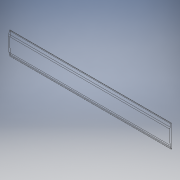
# Autodesk Inventor part: element_1
Saved by Autodesk Inventor 2018.1 (Build 221171000, 171)
## iProperties
Created: 2017-10-22
Part Number: element_1
Material: CFRP
Document SubType Name: Modeling
Designer: ku_sk
Density: 1.43 g/cm^3
Appearance: カーボンファイバー
Mass: 1502.98 g
Surface Area: 2648.54 cm^2
Volume: 1051.04 cm^3
Author: ku_sk
Autodesk Inventor part; units mm, degrees
ref_plane "YZ Plane" through (0, 0, 0) normal (1, 0, 0) x (0, 1, 0)
ref_plane "XZ Plane" through (0, 0, 0) normal (0, 1, 0) x (-1, 0, 0)
ref_plane "XY Plane" through (0, 0, 0) normal (0, 0, 1) x (1, 0, 0)
sketch "スケッチ1" plane through (0, 0, 0) normal (1, 0, 0) x (0, 1, 0)
  line L0 (0, 91.5) -> (0, -91.5)
  line L1 (-146.6441, 0) -> (763.437, 0) projected
  arc A0 (0, 91.5) -> (0, -91.5) centre (633.4254, 0) ccw
  arc A1 (0, 91.5) -> (0, -91.5) centre (243.3675, 0) ccw
  point P0 (0, 0)
  point P1 (0, 0)
  dimension "d0" = 183
  dimension "d1" = 640
  dimension "d2" = 260
  constraints: 4 point on circle, 2 centre point, 2 end point, 2 midpoint, 1 point on line, 1 vertical
  measures "d0" distance of L0.start L0.end
  measures "d1" radius of A0
  measures "d2" radius of A1
extrude "押し出し1" add sketch "スケッチ1" along normal mid plane 950 contours A0 L1 A1 | A0 A1 L1
fillet "フィレット1" radius 3 1 edges at (0, 0, 91.5)
fillet "フィレット2" radius 2 1 edges at (0, 0, -91.5)
sketch "スケッチ2" plane through (475, 0, 0) normal (1, 0, 0) x (0, 0, -1)
  line L0 (-44.0145, -12.8799) -> (-34.1281, -14.3829)
  line L1 (59.0473, -9.8388) -> (49.2667, -11.9221)
  arc A0 (-59.026, -9.8437) -> (71.7475, -6.537) centre (0, 243.3675) ccw projected
  point P0 (0, 0)
  dimension "d7" = 10
  dimension "d8" = 10
  constraints: 4 end point, 4 point on circle
  measures "d7" distance of L0.start L0.end
  measures "d8" distance of L1.start L1.end
extrude "押し出し2" cut sketch "スケッチ2" against normal through all
